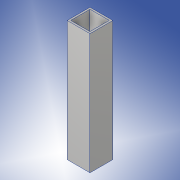
# Autodesk Inventor part: C006
Saved by Autodesk Inventor 2017 (Build 210142000, 142)
## iProperties
Created: 2017-06-14
Part Number: C006
Material: Aluminum 6061
Document SubType Name: Modeling
Designer: zallen
Density: 2.7 g/cm^3
Appearance: Aluminum - Flat
Author: zallen
Autodesk Inventor part; units mm, degrees
ref_plane "YZ Plane" through (0, 0, 0) normal (1, 0, 0) x (0, 1, 0)
ref_plane "XZ Plane" through (0, 0, 0) normal (0, 1, 0) x (-1, 0, 0)
ref_plane "XY Plane" through (0, 0, 0) normal (0, 0, 1) x (1, 0, 0)
sketch "Sketch1" plane through (0, 0, 0) normal (0, 0, 1) x (1, 0, 0)
  line L0 (0, 0) -> (19, 0)
  line L1 (19, 0) -> (19, 100)
  line L2 (19, 100) -> (0, 100)
  line L3 (0, 100) -> (0, 0)
  dimension "d0" = 19
  dimension "d1" = 100
  constraints: 8 end point, 2 parallel, 1 horizontal, 1 perpendicular
  measures "d0" distance of L2.end L1.end
  measures "d1" distance of L1.end L0.end
extrude "Extrusion1" add sketch "Sketch1" along normal blind 19
sketch "Sketch3" plane through (0, 100, 0) normal (0, 1, 0) x (1, 0, 0)
  line L0 (19, 0) -> (0, 0) projected
  line L1 (0, 0) -> (0, -19) projected
  line L2 (19, -19) -> (0, -19) projected
  line L3 (19, 0) -> (19, -19) projected
  line L4 (1.5, -17.5) -> (1.5, -1.5)
  line L5 (1.5, -1.5) -> (17.5, -1.5)
  line L6 (17.5, -1.5) -> (17.5, -17.5)
  line L7 (17.5, -17.5) -> (1.5, -17.5)
  point P0 (0, 0)
  dimension "d4" = 1.5
  constraints: 8 end point, 3 other
  measures "d4" distance between parallel lines of L1 L4
extrude "Extrusion2" cut sketch "Sketch3" against normal through all contours L4 L5 L6 L7
body "Solid1"
